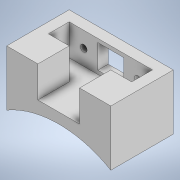
# Autodesk Inventor part: BracketForScope
Saved by Autodesk Inventor 2022.2 (Build 262287000, 287)
## iProperties
Created: 2021-12-26
Part Number: BracketForScope
Material: Generic
Document SubType Name: Modeling
Designer: robst
Density: 1 g/cm^3
Appearance: Default
Author: robst
Autodesk Inventor part; units mm, degrees
ref_plane "YZ Plane" through (0, 0, 0) normal (1, 0, 0) x (0, 1, 0)
ref_plane "XZ Plane" through (0, 0, 0) normal (0, 1, 0) x (-1, 0, 0)
ref_plane "XY Plane" through (0, 0, 0) normal (0, 0, 1) x (1, 0, 0)
sketch "Sketch1" plane through (0, 0, 0) normal (0, 0, 1) x (1, 0, 0)
  arc A0 (25, 43.3013) -> (-25, 43.3013) centre (0, 0) ccw
  line L0 (0, 0) -> (0, 50) construction
  line L1 (0, 50) -> (25, 50)
  line L2 (0, 50) -> (-25, 50)
  line L3 (-25, 50) -> (-25, 43.3013)
  line L4 (25, 50) -> (25, 43.3013)
  line L5 (-25, 50) -> (25, 50)
  line L6 (25, 50) -> (25, 55)
  line L7 (25, 55) -> (-25, 55)
  line L8 (-25, 55) -> (-25, 50)
  dimension "d0" = 100
  dimension "d1" = 50
  dimension "d2" = 5
  constraints: 18 end point, 3 horizontal, 3 parallel, 3 point on circle, 2 vertical, 1 centre point, 1 coincident, 1 collinear, 1 perpendicular, 1 tangent
  measures "d0" diameter of A0
  measures "d1" distance of L1.end L2.end
  measures "d2" distance of L7.end L2.end
extrude "Extrusion1" add sketch "Sketch1" along normal mid plane 30
sketch "Sketch2" plane through (-25, 55, 15) normal (0, 1, 0) x (1, 0, 0)
  line L0 (50, 0) -> (0, 0) construction
  line L1 (25, 0) -> (25, 29.8898) construction
  line L2 (50, 0) -> (0, 0) construction
  line L3 (15, 0) -> (35, 0)
  line L4 (35, 0) -> (35, 15)
  line L5 (35, 15) -> (15, 15)
  line L6 (15, 15) -> (15, 0)
  line L7 (15, 0) -> (35, 15) construction
  line L8 (35, 0) -> (15, 15) construction
  line L9 (5, 15) -> (45, 15)
  line L10 (45, 15) -> (45, 25)
  line L11 (45, 25) -> (5, 25)
  line L12 (5, 25) -> (5, 15)
  line L13 (5, 15) -> (45, 25) construction
  line L14 (45, 15) -> (5, 25) construction
  line L15 (0, 30) -> (50, 30) projected
  line L16 (50, 30) -> (50, 0) projected
  line L17 (0, 0) -> (50, 0)
  line L18 (50, 0) -> (50, 30)
  line L19 (50, 30) -> (0, 30)
  line L20 (0, 30) -> (0, 0)
  point P0 (25, 15)
  point P1 (25, 7.5)
  point P2 (25, 20)
  point P3 (35, 0)
  point P4 (15, 0)
  dimension "d5" = 20
  dimension "d6" = 15
  dimension "d7" = 40
  dimension "d8" = 10
  dimension "d9" = 5
  constraints: 34 end point, 6 parallel, 5 midpoint, 5 perpendicular, 2 collinear, 2 point on line, 1 horizontal, 1 vertical
  measures "d5" distance of L4.end L5.end
  measures "d6" distance of L5.end L3.start
  measures "d7" distance of L10.end L11.end
  measures "d8" distance of L11.end L9.start
  measures "d9" distance between parallel lines of L11 L15
extrude "Extrusion2" add sketch "Sketch2" along normal blind 15 contours L17 L20 L15 L16 L4 L9 L10 L11 L12 L6
sketch "Sketch3" plane through (0, 0, -15) normal (0, 0, -1) x (-1, 0, 0)
  line L0 (-20, 55) -> (20, 55) projected
  line L1 (-25, 70) -> (25, 70) projected
  line L2 (20, 55) -> (20, 70) projected
  line L3 (-20, 55) -> (-20, 70) projected
  line L4 (0, 70) -> (0, 55) construction
  line L5 (20, 55) -> (20, 70) construction
  line L6 (20, 62.5) -> (-20, 62.5) construction
  line L7 (-6.25, 68.25) -> (-6.25, 56.75)
  line L8 (-6.25, 56.75) -> (6.25, 56.75)
  line L9 (6.25, 56.75) -> (6.25, 68.25)
  line L10 (6.25, 68.25) -> (-6.25, 68.25)
  line L11 (-6.25, 68.25) -> (6.25, 56.75) construction
  line L12 (-6.25, 56.75) -> (6.25, 68.25) construction
  point P0 (0, 0)
  point P1 (0, 62.5)
  dimension "d12" = 11.5
  dimension "d13" = 12.5
  constraints: 16 end point, 7 midpoint, 2 parallel, 1 perpendicular, 1 vertical
  measures "d12" distance of L8.end L9.end
  measures "d13" distance of L9.end L7.start
extrude "Extrusion3" cut sketch "Sketch3" against normal up to surface (5 mm away) contours L10 L9 L8 L7
sketch "Sketch5" plane through (0, 0, -15) normal (0, 0, -1) x (-1, 0, 0)
  line L0 (-20, 55) -> (20, 55) projected
  line L1 (20, 55) -> (20, 70) projected
  line L2 (-20, 55) -> (-20, 70) projected
  line L3 (-10, 55) -> (10, 55) construction
  line L4 (0, 55) -> (0, 70) construction
  line L5 (0, 62.5) -> (13, 62.5) construction
  line L6 (0, 62.5) -> (-13, 62.5) construction
  point P0 (0, 0)
  dimension "d16" = 26
  constraints: 6 end point, 2 coincident, 2 horizontal, 2 midpoint, 1 collinear, 1 vertical
  measures "d16" distance of L5.end L6.end
hole "Hole1" at (13, 62.5, -15) at (-13, 62.5, -15) direction (0, 0, 1) diameter 3.264 end up to face face through (-15.4167, 60.5833, -10) facing (0, 0, 1) clearance for "Flat Head Machine Screw (82)" size "#4" standard "Ansi Unified Screw Threads"
body "Solid1"
